Autodesk Fusion 360 part; units mm, degrees
(part 2 of 3)
sketch "Sketch2 (2)" plane through (0, 0, 0) normal (-1, 0, 0) x (0, -1, 0) in component "left"
  line L0 (-22.5, 130) -> (-22.5, 127)
  line L1 (-22.5, 127) -> (-32.1429, 127)
  line L2 (-32.1429, 127) -> (-32.1429, 130)
  line L3 (-32.1429, 130) -> (-42.8571, 130)
  line L4 (-42.8571, 130) -> (-42.8571, 127)
  line L5 (-42.8571, 127) -> (-52.5, 127)
  line L6 (-52.5, 127) -> (-52.5, 130)
  line L7 (-52.5, 130) -> (-52.5, 200)
  line L8 (-52.5, 200) -> (-72, 200)
  line L9 (-72, 200) -> (-72, 177.7778)
  line L10 (-72, 177.7778) -> (-75, 177.7778)
  line L11 (-75, 177.7778) -> (-75, 155.5556)
  line L12 (-75, 155.5556) -> (-72, 155.5556)
  line L13 (-72, 155.5556) -> (-72, 133.3333)
  line L14 (-72, 133.3333) -> (-75, 133.3333)
  line L15 (-75, 133.3333) -> (-75, 111.1111)
  line L16 (-75, 111.1111) -> (-72, 111.1111)
  line L17 (-72, 111.1111) -> (-72, 88.8889)
  line L18 (-72, 88.8889) -> (-75, 88.8889)
  line L19 (-75, 88.8889) -> (-75, 66.6667)
  line L20 (-75, 66.6667) -> (-72, 66.6667)
  line L21 (-72, 66.6667) -> (-72, 44.4444)
  line L22 (-72, 44.4444) -> (-75, 44.4444)
  line L23 (-75, 44.4444) -> (-75, 22.2222)
  line L24 (-75, 22.2222) -> (-72, 22.2222)
  line L25 (-72, 22.2222) -> (-72, 3)
  line L26 (-72, 3) -> (-64.2857, 3)
  line L27 (-64.2857, 3) -> (-64.2857, 0)
  line L28 (-64.2857, 0) -> (-53.5714, 0)
  line L29 (-53.5714, 0) -> (-53.5714, 3)
  line L30 (-53.5714, 3) -> (-42.8571, 3)
  line L31 (-42.8571, 3) -> (-42.8571, 0)
  line L32 (-42.8571, 0) -> (-32.1429, 0)
  line L33 (-32.1429, 0) -> (-32.1429, 3)
  line L34 (-32.1429, 3) -> (-21.4286, 3)
  line L35 (-21.4286, 3) -> (-21.4286, 0)
  line L36 (-21.4286, 0) -> (-10.7143, 0)
  line L37 (-10.7143, 0) -> (-10.7143, 3)
  line L38 (-10.7143, 3) -> (-3, 3)
  line L39 (-3, 3) -> (-3, 22.2222)
  line L40 (-3, 22.2222) -> (0, 22.2222)
  line L41 (0, 22.2222) -> (0, 44.4444)
  line L42 (0, 44.4444) -> (-3, 44.4444)
  line L43 (-3, 44.4444) -> (-3, 66.6667)
  line L44 (-3, 66.6667) -> (0, 66.6667)
  line L45 (0, 66.6667) -> (0, 88.8889)
  line L46 (0, 88.8889) -> (-3, 88.8889)
  line L47 (-3, 88.8889) -> (-3, 111.1111)
  line L48 (-3, 111.1111) -> (0, 111.1111)
  line L49 (0, 111.1111) -> (0, 133.3333)
  line L50 (0, 133.3333) -> (-3, 133.3333)
  line L51 (-3, 133.3333) -> (-3, 155.5556)
  line L52 (-3, 155.5556) -> (0, 155.5556)
  line L53 (0, 155.5556) -> (0, 177.7778)
  line L54 (0, 177.7778) -> (-3, 177.7778)
  line L55 (-3, 177.7778) -> (-3, 200)
  line L56 (-3, 200) -> (-22.5, 200)
  line L57 (-22.5, 200) -> (-22.5, 130)
  line L58 (-52.5, 200) -> (-22.5, 200)
  line L59 (-22.5, 200) -> (-22.5, 156)
  line L60 (-22.5, 156) -> (-52.5, 156)
  line L61 (-52.5, 156) -> (-52.5, 200)
  dimension "d161" = 26
  constraint horizontal L58
  constraint vertical L59
  constraint horizontal L60
  constraint vertical L61
  constraint coincident L57 L59.end
  constraint coincident L7.end L8.start
  measures "d161" distance of L3 L60
extrude "Extrude4'''" add sketch "Sketch2 (2)" against normal blind 3 contours L7 L57 L58 L59 L60 L61 bodies 5 in component "left"
combine "Combine6" operation cut target body 4 tool bodies 8 keep tools in component "right"
sketch "Sketch3 (2)" plane through (0, 0, 0) normal (-1, 0, 0) x (0, -1, 0) in component "left"
  line L0 (-22.5, 156) -> (-22.5, 130)
  line L1 (-22.5, 130) -> (-22.5, 127)
  line L2 (-22.5, 127) -> (-32.1429, 127)
  line L3 (-32.1429, 127) -> (-32.1429, 130)
  line L4 (-32.1429, 130) -> (-42.8571, 130)
  line L5 (-42.8571, 130) -> (-42.8571, 127)
  line L6 (-42.8571, 127) -> (-52.5, 127)
  line L7 (-52.5, 127) -> (-52.5, 130)
  line L8 (-52.5, 130) -> (-52.5, 156)
  line L9 (-52.5, 156) -> (-22.5, 156)
  line L10 (-3, 200) -> (-72, 200)
  line L11 (-72, 200) -> (-72, 177.7778)
  line L12 (-72, 177.7778) -> (-75, 177.7778)
  line L13 (-75, 177.7778) -> (-75, 155.5556)
  line L14 (-75, 155.5556) -> (-72, 155.5556)
  line L15 (-72, 155.5556) -> (-72, 133.3333)
  line L16 (-72, 133.3333) -> (-75, 133.3333)
  line L17 (-75, 133.3333) -> (-75, 111.1111)
  line L18 (-75, 111.1111) -> (-72, 111.1111)
  line L19 (-72, 111.1111) -> (-72, 88.8889)
  line L20 (-72, 88.8889) -> (-75, 88.8889)
  line L21 (-75, 88.8889) -> (-75, 66.6667)
  line L22 (-75, 66.6667) -> (-72, 66.6667)
  line L23 (-72, 66.6667) -> (-72, 44.4444)
  line L24 (-72, 44.4444) -> (-75, 44.4444)
  line L25 (-75, 44.4444) -> (-75, 22.2222)
  line L26 (-75, 22.2222) -> (-72, 22.2222)
  line L27 (-72, 22.2222) -> (-72, 3)
  line L28 (-72, 3) -> (-64.2857, 3)
  line L29 (-64.2857, 3) -> (-64.2857, 0)
  line L30 (-64.2857, 0) -> (-53.5714, 0)
  line L31 (-53.5714, 0) -> (-53.5714, 3)
  line L32 (-53.5714, 3) -> (-42.8571, 3)
  line L33 (-42.8571, 3) -> (-42.8571, 0)
  line L34 (-42.8571, 0) -> (-32.1429, 0)
  line L35 (-32.1429, 0) -> (-32.1429, 3)
  line L36 (-32.1429, 3) -> (-21.4286, 3)
  line L37 (-21.4286, 3) -> (-21.4286, 0)
  line L38 (-21.4286, 0) -> (-10.7143, 0)
  line L39 (-10.7143, 0) -> (-10.7143, 3)
  line L40 (-10.7143, 3) -> (-3, 3)
  line L41 (-3, 3) -> (-3, 22.2222)
  line L42 (-3, 22.2222) -> (0, 22.2222)
  line L43 (0, 22.2222) -> (0, 44.4444)
  line L44 (0, 44.4444) -> (-3, 44.4444)
  line L45 (-3, 44.4444) -> (-3, 66.6667)
  line L46 (-3, 66.6667) -> (0, 66.6667)
  line L47 (0, 66.6667) -> (0, 88.8889)
  line L48 (0, 88.8889) -> (-3, 88.8889)
  line L49 (-3, 88.8889) -> (-3, 111.1111)
  line L50 (-3, 111.1111) -> (0, 111.1111)
  line L51 (0, 111.1111) -> (0, 133.3333)
  line L52 (0, 133.3333) -> (-3, 133.3333)
  line L53 (-3, 133.3333) -> (-3, 155.5556)
  line L54 (-3, 155.5556) -> (0, 155.5556)
  line L55 (0, 155.5556) -> (0, 177.7778)
  line L56 (0, 177.7778) -> (-3, 177.7778)
  line L57 (-3, 177.7778) -> (-3, 200)
  circle A0 centre (-60, 117) radius 2.5
  dimension "d164" = 10
  dimension "d165" = 5
  dimension "d166" = 15
  measures "d164" distance of L6 A0.centre
  measures "d165" diameter of A0
  measures "d166" distance of L17 A0.centre
extrude "Extrude5'''" cut sketch "Sketch3 (2)" against normal blind 3 contours A0 bodies 5 in component "left"
sketch "Sketch7" plane through (75, 0, 0) normal (1, 0, 0) x (0, 1, 0) in component "right"
  line L0 (72, 78) -> (72, 66.6667)
  line L1 (72, 66.6667) -> (75, 66.6667)
  line L2 (75, 66.6667) -> (75, 88.8889)
  line L3 (75, 88.8889) -> (72, 88.8889)
  line L4 (72, 88.8889) -> (72, 111.1111)
  line L5 (72, 111.1111) -> (75, 111.1111)
  line L6 (75, 111.1111) -> (75, 133.3333)
  line L7 (75, 133.3333) -> (72, 133.3333)
  line L8 (72, 133.3333) -> (72, 155.5556)
  line L9 (72, 155.5556) -> (75, 155.5556)
  line L10 (75, 155.5556) -> (75, 177.7778)
  line L11 (75, 177.7778) -> (72, 177.7778)
  line L12 (72, 177.7778) -> (72, 200)
  line L13 (72, 200) -> (3, 200)
  line L14 (3, 200) -> (3, 177.7778)
  line L15 (3, 177.7778) -> (0, 177.7778)
  line L16 (0, 177.7778) -> (0, 155.5556)
  line L17 (0, 155.5556) -> (3, 155.5556)
  line L18 (3, 155.5556) -> (3, 133.3333)
  line L19 (3, 133.3333) -> (0, 133.3333)
  line L20 (0, 133.3333) -> (0, 111.1111)
  line L21 (0, 111.1111) -> (3, 111.1111)
  line L22 (3, 111.1111) -> (3, 88.8889)
  line L23 (3, 88.8889) -> (0, 88.8889)
  line L24 (0, 88.8889) -> (0, 66.6667)
  line L25 (0, 66.6667) -> (3, 66.6667)
  line L26 (3, 66.6667) -> (3, 44.4444)
  line L27 (3, 44.4444) -> (0, 44.4444)
  line L28 (0, 44.4444) -> (0, 22.2222)
  line L29 (0, 22.2222) -> (3, 22.2222)
  line L30 (3, 22.2222) -> (3, 3)
  line L31 (3, 3) -> (10.7143, 3)
  line L32 (10.7143, 3) -> (10.7143, 0)
  line L33 (10.7143, 0) -> (21.4286, 0)
  line L34 (21.4286, 0) -> (21.4286, 3)
  line L35 (21.4286, 3) -> (32.1429, 3)
  line L36 (32.1429, 3) -> (32.1429, 0)
  line L37 (32.1429, 0) -> (42.8571, 0)
  line L38 (42.8571, 0) -> (42.8571, 3)
  line L39 (42.8571, 3) -> (53.5714, 3)
  line L40 (53.5714, 3) -> (53.5714, 0)
  line L41 (53.5714, 0) -> (64.2857, 0)
  line L42 (64.2857, 0) -> (64.2857, 3)
  line L43 (64.2857, 3) -> (69, 3)
  line L44 (69, 3) -> (69, 78)
  line L45 (69, 78) -> (72, 78)
  circle A0 centre (60, 117) radius 2.5
  line L46 (52.5, 127) -> (42.8571, 127)
  line L47 (75, 0) -> (75, 200)
  dimension "d171" = 5
  dimension "d190" = 10
  dimension "d191" = 15
  measures "d171" diameter of A0
  measures "d190" distance of A0.centre L46
  measures "d191" distance of A0.centre L47
extrude "Extrude8" cut sketch "Sketch7" against normal blind 8 contours A0 bodies 4 in component "right"
sketch "Sketch3 (3)" plane through (0, 0, 0) normal (0, -1, 0) x (1, 0, 0) in component "front"
  line L0 (52.5, 156) -> (52.5, 130)
  line L1 (52.5, 130) -> (50, 130)
  line L2 (50, 130) -> (50, 127)
  line L3 (50, 127) -> (41.6667, 127)
  line L4 (41.6667, 127) -> (41.6667, 130)
  line L5 (41.6667, 130) -> (33.3333, 130)
  line L6 (33.3333, 130) -> (33.3333, 127)
  line L7 (33.3333, 127) -> (25, 127)
  line L8 (25, 127) -> (25, 130)
  line L9 (25, 130) -> (22.5, 130)
  line L10 (22.5, 130) -> (22.5, 156)
  line L11 (22.5, 156) -> (52.5, 156)
  line L12 (75, 200) -> (0, 200)
  line L13 (0, 200) -> (0, 177.7778)
  line L14 (0, 177.7778) -> (3, 177.7778)
  line L15 (3, 177.7778) -> (3, 155.5556)
  line L16 (3, 155.5556) -> (0, 155.5556)
  line L17 (0, 155.5556) -> (0, 133.3333)
  line L18 (0, 133.3333) -> (3, 133.3333)
  line L19 (3, 133.3333) -> (3, 111.1111)
  line L20 (3, 111.1111) -> (0, 111.1111)
  line L21 (0, 111.1111) -> (0, 88.8889)
  line L22 (0, 88.8889) -> (3, 88.8889)
  line L23 (3, 88.8889) -> (3, 66.6667)
  line L24 (3, 66.6667) -> (0, 66.6667)
  line L25 (0, 66.6667) -> (0, 44.4444)
  line L26 (0, 44.4444) -> (3, 44.4444)
  line L27 (3, 44.4444) -> (3, 22.2222)
  line L28 (3, 22.2222) -> (0, 22.2222)
  line L29 (0, 22.2222) -> (0, 3)
  line L30 (0, 3) -> (8.3333, 3)
  line L31 (8.3333, 3) -> (8.3333, 0)
  line L32 (8.3333, 0) -> (16.6667, 0)
  line L33 (16.6667, 0) -> (16.6667, 3)
  line L34 (16.6667, 3) -> (25, 3)
  line L35 (25, 3) -> (25, 0)
  line L36 (25, 0) -> (33.3333, 0)
  line L37 (33.3333, 0) -> (33.3333, 3)
  line L38 (33.3333, 3) -> (41.6667, 3)
  line L39 (41.6667, 3) -> (41.6667, 0)
  line L40 (41.6667, 0) -> (50, 0)
  line L41 (50, 0) -> (50, 3)
  line L42 (50, 3) -> (58.3333, 3)
  line L43 (58.3333, 3) -> (58.3333, 0)
  line L44 (58.3333, 0) -> (66.6667, 0)
  line L45 (66.6667, 0) -> (66.6667, 3)
  line L46 (66.6667, 3) -> (75, 3)
  line L47 (75, 3) -> (75, 22.2222)
  line L48 (75, 22.2222) -> (72, 22.2222)
  line L49 (72, 22.2222) -> (72, 44.4444)
  line L50 (72, 44.4444) -> (75, 44.4444)
  line L51 (75, 44.4444) -> (75, 66.6667)
  line L52 (75, 66.6667) -> (72, 66.6667)
  line L53 (72, 66.6667) -> (72, 88.8889)
  line L54 (72, 88.8889) -> (75, 88.8889)
  line L55 (75, 88.8889) -> (75, 111.1111)
  line L56 (75, 111.1111) -> (72, 111.1111)
  line L57 (72, 111.1111) -> (72, 133.3333)
  line L58 (72, 133.3333) -> (75, 133.3333)
  line L59 (75, 133.3333) -> (75, 155.5556)
  line L60 (75, 155.5556) -> (72, 155.5556)
  line L61 (72, 155.5556) -> (72, 177.7778)
  line L62 (72, 177.7778) -> (75, 177.7778)
  line L63 (75, 177.7778) -> (75, 200)
  circle A0 centre (18, 117) radius 2.5
  dimension "d174" = 10
  dimension "d175" = 15
  dimension "d176" = 5
  measures "d174" distance of L7 A0.centre
  measures "d175" distance of L19 A0.centre
  measures "d176" diameter of A0
extrude "Extrude5''''" cut sketch "Sketch3 (3)" against normal blind 3 contours A0 bodies 3 in component "front"
sketch "Sketch6 (2)" plane through (0, 72, 0) normal (0, -1, 0) x (1, 0, 0) in component "back"
  line L0 (13, 8) -> (13, 78)
  line L1 (13, 78) -> (62, 78)
  line L2 (62, 78) -> (62, 8)
  line L3 (62, 8) -> (13, 8)
  line L4 (0, 3) -> (8.3333, 3)
  line L5 (8.3333, 3) -> (8.3333, 0)
  line L6 (8.3333, 0) -> (16.6667, 0)
  line L7 (16.6667, 0) -> (16.6667, 3)
  line L8 (16.6667, 3) -> (25, 3)
  line L9 (25, 3) -> (25, 0)
  line L10 (25, 0) -> (33.3333, 0)
  line L11 (33.3333, 0) -> (33.3333, 3)
  line L12 (33.3333, 3) -> (41.6667, 3)
  line L13 (41.6667, 3) -> (41.6667, 0)
  line L14 (41.6667, 0) -> (50, 0)
  line L15 (50, 0) -> (50, 3)
  line L16 (50, 3) -> (58.3333, 3)
  line L17 (58.3333, 3) -> (58.3333, 0)
  line L18 (58.3333, 0) -> (66.6667, 0)
  line L19 (66.6667, 0) -> (66.6667, 3)
  line L20 (66.6667, 3) -> (75, 3)
  line L21 (75, 3) -> (75, 22.2222)
  line L22 (75, 22.2222) -> (75, 44.4444)
  line L23 (75, 44.4444) -> (75, 66.6667)
  line L24 (75, 66.6667) -> (72, 66.6667)
  line L25 (72, 66.6667) -> (72, 88.8889)
  line L26 (72, 88.8889) -> (75, 88.8889)
  line L27 (75, 88.8889) -> (75, 111.1111)
  line L28 (75, 111.1111) -> (72, 111.1111)
  line L29 (72, 111.1111) -> (72, 133.3333)
  line L30 (72, 133.3333) -> (75, 133.3333)
  line L31 (75, 133.3333) -> (75, 155.5556)
  line L32 (75, 155.5556) -> (72, 155.5556)
  line L33 (72, 155.5556) -> (72, 177.7778)
  line L34 (72, 177.7778) -> (75, 177.7778)
  line L35 (75, 177.7778) -> (75, 200)
  line L36 (75, 200) -> (0, 200)
  line L37 (0, 200) -> (0, 177.7778)
  line L38 (0, 177.7778) -> (3, 177.7778)
  line L39 (3, 177.7778) -> (3, 155.5556)
  line L40 (3, 155.5556) -> (0, 155.5556)
  line L41 (0, 155.5556) -> (0, 133.3333)
  line L42 (0, 133.3333) -> (3, 133.3333)
  line L43 (3, 133.3333) -> (3, 111.1111)
  line L44 (3, 111.1111) -> (0, 111.1111)
  line L45 (0, 111.1111) -> (0, 88.8889)
  line L46 (0, 88.8889) -> (3, 88.8889)
  line L47 (3, 88.8889) -> (3, 66.6667)
  line L48 (3, 66.6667) -> (0, 66.6667)
  line L49 (0, 66.6667) -> (0, 44.4444)
  line L50 (0, 44.4444) -> (3, 44.4444)
  line L51 (3, 44.4444) -> (3, 22.2222)
  line L52 (3, 22.2222) -> (0, 22.2222)
  line L53 (0, 22.2222) -> (0, 3)
  circle A0 centre (37.5, 117) radius 2.5
  line L54 (3, 127) -> (72, 127)
  line L55 (37.5, 117) -> (37.5, 127)
  dimension "d183" = 5
  dimension "d186" = 10
  constraint coincident A0.centre L55.start
  constraint coincident L54 L55.end
  constraint perpendicular L54 L55
  constraint midpoint L54 L55.end
  measures "d183" diameter of A0
  measures "d186" distance of A0.centre L55.end
extrude "Extrude7'" cut sketch "Sketch6 (2)" against normal blind 6 contours A0 bodies 2 in component "back"
extrude "Extrude9" cut sketch "spout_cut" against normal blind 10 contours L30 L48 L49 L50 L51 bodies 4 in component "right"
sketch "Sketch8" plane through (75, 0, 0) normal (1, 0, 0) x (0, 1, 0) in component "right"
  line L0 (52.5, 156) -> (22.5, 156)
  line L1 (22.5, 156) -> (22.5, 200)
  line L2 (22.5, 200) -> (52.5, 200)
  line L3 (52.5, 200) -> (52.5, 156)
  line L4 (22.5, 156) -> (52.5, 156)
  line L5 (52.5, 200) -> (52.5, 130)
  point P0 (22.5, 200)
  constraint horizontal L0
  constraint vertical L1
  constraint horizontal L2
  constraint vertical L3
  constraint coincident P0 L1.end
  constraint coincident L0.start L4
  constraint coincident L2.end L5
extrude "Extrude10" add sketch "Sketch8" against normal blind 3 bodies 4 in component "right"
combine "Combine7" operation cut target body 4 tool bodies 6 keep tools in component "right"
sketch "Sketch1 (5)" plane through (0, 0, 200) normal (0, 0, 1) x (-1, 0, 0) in component "cover"
  line L0 (-75, -75) -> (0, -75)
  line L1 (0, -75) -> (0, -72)
  line L2 (0, -72) -> (-75, -72)
  line L3 (-75, -72) -> (-75, -75)
  line L4 (-75, -75) -> (0, -75)
  line L5 (0, -75) -> (0, 0)
  line L6 (0, 0) -> (-75, 0)
  line L7 (-75, 0) -> (-75, -75)
  line L8 (5, 5) -> (-80, 5)
  line L9 (-80, 5) -> (-80, -80)
  line L10 (-80, -80) -> (5, -80)
  line L11 (5, -80) -> (5, 5)
  line L12 (0, -64.2857) -> (-3, -64.2857)
  line L13 (-3, -64.2857) -> (-3, -53.5714)
  line L14 (-3, -53.5714) -> (0, -53.5714)
  line L15 (0, -53.5714) -> (0, -64.2857)
  line L16 (0, -64.2857) -> (-3, -64.2857)
  line L17 (-3, -53.5714) -> (0, -53.5714)
  line L18 (-3, -42.8571) -> (0, -42.8571)
  line L19 (0, -42.8571) -> (0, -32.1429)
  line L20 (0, -32.1429) -> (-3, -32.1429)
  line L21 (-3, -32.1429) -> (-3, -42.8571)
  line L22 (-3, -21.4286) -> (0, -21.4286)
  line L23 (0, -21.4286) -> (0, -10.7143)
  line L24 (0, -10.7143) -> (-3, -10.7143)
  line L25 (-3, -10.7143) -> (-3, -21.4286)
  line L26 (0, -21.4286) -> (-3, -21.4286)
  line L27 (-3, -32.1429) -> (0, -32.1429)
  line L28 (-16.6667, -75) -> (-8.3333, -75)
  line L29 (-8.3333, -75) -> (-8.3333, -72)
  line L30 (-8.3333, -72) -> (-16.6667, -72)
  line L31 (-16.6667, -72) -> (-16.6667, -75)
  line L32 (-33.3333, -75) -> (-25, -75)
  line L33 (-25, -75) -> (-25, -72)
  line L34 (-25, -72) -> (-33.3333, -72)
  line L35 (-33.3333, -72) -> (-33.3333, -75)
  line L36 (-50, -75) -> (-41.6667, -75)
  line L37 (-41.6667, -75) -> (-41.6667, -72)
  line L38 (-41.6667, -72) -> (-50, -72)
  line L39 (-50, -72) -> (-50, -75)
  line L40 (-66.6667, -75) -> (-58.3333, -75)
  line L41 (-58.3333, -75) -> (-58.3333, -72)
  line L42 (-58.3333, -72) -> (-66.6667, -72)
  line L43 (-66.6667, -72) -> (-66.6667, -75)
  line L44 (-8.3333, -72) -> (-8.3333, -75)
  line L45 (-16.6667, -75) -> (-16.6667, -72)
  line L46 (-25, -72) -> (-25, -75)
  line L47 (-33.3333, -75) -> (-33.3333, -72)
  line L48 (-41.6667, -72) -> (-41.6667, -75)
  line L49 (-58.3333, -72) -> (-58.3333, -75)
  line L50 (-66.6667, -75) -> (-66.6667, -72)
  line L51 (5, -37.5) -> (-80, -37.5) construction
  line L52 (-37.5, -80) -> (-37.5, 5) construction
  line L53 (-72, -42.8571) -> (-75, -42.8571)
  line L54 (-75, -21.4286) -> (-75, -10.7143)
  line L55 (-72, -64.2857) -> (-72, -53.5714)
  line L56 (-75, -64.2857) -> (-72, -64.2857)
  line L57 (-72, -32.1429) -> (-72, -42.8571)
  line L58 (-75, -42.8571) -> (-75, -32.1429)
  line L59 (-72, -53.5714) -> (-75, -53.5714)
  line L60 (-75, -64.2857) -> (-72, -64.2857)
  line L61 (-72, -32.1429) -> (-75, -32.1429)
  line L62 (-75, -32.1429) -> (-72, -32.1429)
  line L63 (-75, -10.7143) -> (-72, -10.7143)
  line L64 (-72, -53.5714) -> (-75, -53.5714)
  line L65 (-75, -75) -> (-75, 0)
  line L66 (-75, -53.5714) -> (-75, -64.2857)
  line L67 (-80, -37.5) -> (5, -37.5) construction
  line L68 (-72, -10.7143) -> (-72, -21.4286)
  line L69 (-72, -21.4286) -> (-75, -21.4286)
  line L70 (-75, -21.4286) -> (-72, -21.4286)
  line L71 (-16.6667, -3) -> (-16.6667, 0)
  line L72 (-16.6667, 0) -> (-8.3333, 0)
  line L73 (-33.3333, -3) -> (-33.3333, 0)
  line L74 (-50, 0) -> (-41.6667, 0)
  line L75 (-8.3333, -3) -> (-16.6667, -3)
  line L76 (-41.6667, -3) -> (-50, -3)
  line L77 (-58.3333, 0) -> (-58.3333, -3)
  line L78 (-41.6667, -3) -> (-41.6667, 0)
  line L79 (-58.3333, -3) -> (-66.6667, -3)
  line L80 (-33.3333, 0) -> (-25, 0)
  line L81 (-25, 0) -> (-25, -3)
  line L82 (-8.3333, 0) -> (-8.3333, -3)
  line L83 (-8.3333, -3) -> (-8.3333, 0)
  line L84 (-66.6667, -3) -> (-66.6667, 0)
  line L85 (-66.6667, 0) -> (-58.3333, 0)
  line L86 (-25, -3) -> (-25, 0)
  line L87 (-66.6667, 0) -> (-66.6667, -3)
  line L88 (-25, -3) -> (-33.3333, -3)
  line L89 (-58.3333, -3) -> (-58.3333, 0)
  line L90 (-41.6667, 0) -> (-41.6667, -3)
  line L91 (-16.6667, 0) -> (-16.6667, -3)
  line L92 (-50, -3) -> (-50, 0)
  line L93 (-33.3333, 0) -> (-33.3333, -3)
  point P0 (-3, -42.8571)
  point P1 (-3, -10.7143)
  point P2 (-50, -72)
  point P3 (-72, -42.8571)
  point P4 (-72, -10.7143)
  point P5 (-50, -3)
  dimension "d199" = 5
  constraint horizontal L4
  constraint vertical L5
  constraint horizontal L6
  constraint vertical L7
  constraint coincident L5.end L6.start
  constraint coincident L0.start L3.end
  constraint horizontal L12
  constraint vertical L13
  constraint horizontal L14
  constraint vertical L15
  constraint coincident L5 L12.start
  constraint coincident L12.end L16
  constraint coincident L13.end L17
  constraint horizontal L18
  constraint vertical L19
  constraint horizontal L20
  constraint vertical L21
  constraint horizontal L22
  constraint vertical L23
  constraint horizontal L24
  constraint vertical L25
  constraint coincident L5 L23.end
  constraint coincident L22.start L26
  constraint coincident L20.end L27
  constraint coincident P0 L18.start
  constraint coincident L13 L12.end
  constraint coincident P1 L24.end
  constraint horizontal L28
  constraint vertical L29
  constraint horizontal L30
  constraint vertical L31
  constraint coincident L2 L29.end
  constraint coincident L4 L28.start
  constraint horizontal L32
  constraint vertical L33
  constraint horizontal L34
  constraint vertical L35
  constraint coincident L2 L33.end
  constraint coincident L4 L32.start
  constraint horizontal L36
  constraint vertical L37
  constraint horizontal L38
  constraint vertical L39
  constraint coincident L2 L37.end
  constraint coincident L4 L36.start
  constraint horizontal L40
  constraint vertical L41
  constraint horizontal L42
  constraint vertical L43
  constraint coincident L2 L41.end
  constraint coincident L4 L40.start
  constraint coincident L29.end L44
  constraint coincident L30.end L45
  constraint coincident L33.end L46
  constraint coincident L34.end L47
  constraint coincident L37.end L48
  constraint coincident L39 P2
  constraint coincident L41.end L49
  constraint coincident L42.end L50
  constraint midpoint L11 L51.start
  constraint midpoint L9 L51.end
  constraint midpoint L10 L52.start
  constraint midpoint L8 L52.end
  constraint symmetric L0.end L52 L0.start
  constraint symmetric L5.end L52 L6.end
  constraint symmetric L12.start L52 L56.start
  constraint symmetric L12.end L52 L55.start
  constraint symmetric L13.end L52 L55.end
  constraint symmetric L14.end L52 L59.end
  constraint symmetric P0 L52 P3
  constraint symmetric L18.end L52 L53.end
  constraint symmetric L19.end L52 L58.end
  constraint symmetric L20.end L52 L57.start
  constraint symmetric L22.start L52 L68.end
  constraint symmetric L22.end L52 L54.start
  constraint symmetric L23.end L52 L54.end
  constraint symmetric P1 L52 P4
  constraint symmetric L51.start L52 L51.end
  constraint symmetric L51.end L52 L51.start
  constraint symmetric L28.start L51 L71.end
  constraint symmetric L28.end L51 L72.end
  constraint symmetric L29.end L51 L75.start
  constraint symmetric L30.end L51 L71.start
  constraint symmetric L32.start L51 L73.end
  constraint symmetric L32.end L51 L80.end
  constraint symmetric L33.end L51 L81.end
  constraint symmetric L34.end L51 L73.start
  constraint symmetric L36.start L51 L74.start
  constraint symmetric L36.end L51 L74.end
  constraint symmetric L37.end L51 L76.start
  constraint symmetric P2 L51 P5
  constraint symmetric L40.start L51 L84.end
  constraint symmetric L40.end L51 L77.start
  constraint symmetric L41.end L51 L77.end
  constraint symmetric L42.end L51 L79.end
extrude "Extrude1'''''''" add sketch "Sketch1 (5)" against normal blind 3 separate body contours L0 L2 L3 L4 L7 L43 L50 L65 | L2 L5 L6 L7 L12 L13 L14 L16 L17 L18 L20 L21 L22 L24 L25 L26 L27 L30 L34 L38 L42 L53 L55 L56 L57 L59 L60 L61 L62 L63 L64 L65 L68 L69 L70 L71 L73 L75 L76 L77 L78 L79 L81 L82 L83 L84 L86 L87 L88 L89 L90 L91 L92 L93 | L0 L2 L4 L39 L41 L49 | L0 L2 L4 L35 L37 L47 L48 | L0 L2 L4 L31 L33 L45 L46 | L0 L1 L2 L4 L5 L29 L44 | L8 L9 L10 L11 makes body 9 in component "cover"
combine "Combine5'" operation cut target body 3 tool bodies 9 keep tools in component "front"
combine "Combine9" operation cut target body 4 tool bodies 9 keep tools in component "right"
combine "Combine5''" operation cut target body 2 tool bodies 9 keep tools in component "back"
combine "Combine4'" operation cut target body 5 tool bodies 9 keep tools in component "left"
sketch "Sketch7 (2)" plane through (0, 75, 0) normal (0, 1, 0) x (-1, 0, 0) in component "back"
  line L0 (-13, 78) -> (-13, 8)
  line L1 (-13, 8) -> (-62, 8)
  line L2 (-62, 8) -> (-62, 78)
  line L3 (-62, 78) -> (-13, 78)
  circle A0 centre (-37.5, 117) radius 2.5
  line L4 (0, 197) -> (-8.3333, 197)
  line L5 (-8.3333, 197) -> (-8.3333, 200)
  line L6 (-8.3333, 200) -> (-16.6667, 200)
  line L7 (-16.6667, 200) -> (-16.6667, 197)
  line L8 (-16.6667, 197) -> (-25, 197)
  line L9 (-25, 197) -> (-25, 200)
  line L10 (-25, 200) -> (-33.3333, 200)
  line L11 (-33.3333, 200) -> (-33.3333, 197)
  line L12 (-33.3333, 197) -> (-41.6667, 197)
  line L13 (-41.6667, 197) -> (-41.6667, 200)
  line L14 (-41.6667, 200) -> (-50, 200)
  line L15 (-50, 200) -> (-50, 197)
  line L16 (-50, 197) -> (-58.3333, 197)
  line L17 (-58.3333, 197) -> (-58.3333, 200)
  line L18 (-58.3333, 200) -> (-66.6667, 200)
  line L19 (-66.6667, 200) -> (-66.6667, 197)
  line L20 (-66.6667, 197) -> (-75, 197)
  line L21 (-75, 197) -> (-75, 177.7778)
  line L22 (-75, 177.7778) -> (-72, 177.7778)
  line L23 (-72, 177.7778) -> (-72, 155.5556)
  line L24 (-72, 155.5556) -> (-75, 155.5556)
  line L25 (-75, 155.5556) -> (-75, 133.3333)
  line L26 (-75, 133.3333) -> (-72, 133.3333)
  line L27 (-72, 133.3333) -> (-72, 111.1111)
  line L28 (-72, 111.1111) -> (-75, 111.1111)
  line L29 (-75, 111.1111) -> (-75, 88.8889)
  line L30 (-75, 88.8889) -> (-72, 88.8889)
  line L31 (-72, 88.8889) -> (-72, 66.6667)
  line L32 (-72, 66.6667) -> (-75, 66.6667)
  line L33 (-75, 66.6667) -> (-75, 44.4444)
  line L34 (-75, 44.4444) -> (-75, 22.2222)
  line L35 (-75, 22.2222) -> (-75, 3)
  line L36 (-75, 3) -> (-66.6667, 3)
  line L37 (-66.6667, 3) -> (-66.6667, 0)
  line L38 (-66.6667, 0) -> (-58.3333, 0)
  line L39 (-58.3333, 0) -> (-58.3333, 3)
  line L40 (-58.3333, 3) -> (-50, 3)
  line L41 (-50, 3) -> (-50, 0)
  line L42 (-50, 0) -> (-41.6667, 0)
  line L43 (-41.6667, 0) -> (-41.6667, 3)
  line L44 (-41.6667, 3) -> (-33.3333, 3)
  line L45 (-33.3333, 3) -> (-33.3333, 0)
  line L46 (-33.3333, 0) -> (-25, 0)
  line L47 (-25, 0) -> (-25, 3)
  line L48 (-25, 3) -> (-16.6667, 3)
  line L49 (-16.6667, 3) -> (-16.6667, 0)
  line L50 (-16.6667, 0) -> (-8.3333, 0)
  line L51 (-8.3333, 0) -> (-8.3333, 3)
  line L52 (-8.3333, 3) -> (0, 3)
  line L53 (0, 3) -> (0, 22.2222)
  line L54 (0, 22.2222) -> (-3, 22.2222)
  line L55 (-3, 22.2222) -> (-3, 44.4444)
  line L56 (-3, 44.4444) -> (0, 44.4444)
  line L57 (0, 44.4444) -> (0, 66.6667)
  line L58 (0, 66.6667) -> (-3, 66.6667)
  line L59 (-3, 66.6667) -> (-3, 88.8889)
  line L60 (-3, 88.8889) -> (0, 88.8889)
  line L61 (0, 88.8889) -> (0, 111.1111)
  line L62 (0, 111.1111) -> (-3, 111.1111)
  line L63 (-3, 111.1111) -> (-3, 133.3333)
  line L64 (-3, 133.3333) -> (0, 133.3333)
  line L65 (0, 133.3333) -> (0, 155.5556)
  line L66 (0, 155.5556) -> (-3, 155.5556)
  line L67 (-3, 155.5556) -> (-3, 177.7778)
  line L68 (-3, 177.7778) -> (0, 177.7778)
  line L69 (0, 177.7778) -> (0, 197)
  circle A1 centre (-37.5, 182) radius 5
  line L70 (-37.5, 197) -> (-37.5, 167)
  dimension "d202" = 10
  dimension "d203" = 15
  constraint midpoint L12 L70.start
  constraint perpendicular L12 L70
  constraint coincident A1.centre L70
  measures "d202" diameter of A1
  measures "d203" distance of L12 A1.centre
extrude "Extrude8'" cut sketch "Sketch7 (2)" against normal blind 6 contours A1 L70 | A1 L70 bodies 2 in component "back"
sketch "Sketch1 (6)" plane through (0, 0, 156) normal (0, 0, -1) x (1, 0, 0) in component "Main"
  line L0 (52.5, 0) -> (22.5, 0)
  line L1 (22.5, 0) -> (22.5, -3)
  line L2 (22.5, -3) -> (52.5, -3)
  line L3 (52.5, -3) -> (52.5, 0)
  line L4 (3, -3) -> (72, -3)
  line L5 (72, -3) -> (72, -72)
  line L6 (72, -72) -> (3, -72)
  line L7 (3, -72) -> (3, -3)
  point P0 (3, -3)
  point P1 (66.6667, -72)
  dimension "d206" = 69
  constraint horizontal L4
  constraint vertical L5
  constraint horizontal L6
  constraint vertical L7
  constraint coincident P0 L4.start
  constraint coincident L6 P1
  measures "d206" distance of P0 L4.end
extrude "Extrude1''''''''" add sketch "Sketch1 (6)" against normal blind 2 separate body contours L2 L4 L5 L6 L7 makes body 10 in component "Main"
sketch "Sketch2 (3)" plane through (0, 0, 158) normal (0, 0, 1) x (-1, 0, 0) in component "Main"
  line L0 (-72, -72) -> (-3, -72)
  line L1 (-3, -72) -> (-3, -3)
  line L2 (-3, -3) -> (-72, -3)
  line L3 (-72, -3) -> (-72, -72)
  line L4 (-37.5, -72) -> (-37.5, -3) construction
  line L5 (-3, -37.5) -> (-72, -37.5) construction
  line L6 (-31, -48.875) -> (-44, -48.875)
  line L7 (-44, -48.875) -> (-44, -26.125)
  line L8 (-44, -26.125) -> (-31, -26.125)
  line L9 (-31, -26.125) -> (-31, -48.875)
  line L10 (-31, -48.875) -> (-44, -26.125) construction
  line L11 (-44, -48.875) -> (-31, -26.125) construction
  line L12 (-22, -49.5) -> (-3, -49.5)
  line L13 (-3, -49.5) -> (-3, -25.5)
  line L14 (-3, -25.5) -> (-22, -25.5)
  line L15 (-22, -25.5) -> (-22, -49.5)
  line L16 (-17, -55.875) -> (-58, -55.875)
  line L17 (-58, -55.875) -> (-58, -72)
  line L18 (-58, -72) -> (-17, -72)
  line L19 (-17, -72) -> (-17, -55.875)
  line L20 (-72, -49.5) -> (-53, -49.5)
  line L21 (-53, -49.5) -> (-53, -25.5)
  line L22 (-53, -25.5) -> (-72, -25.5)
  line L23 (-72, -25.5) -> (-72, -49.5)
  line L24 (-49.5, -3) -> (-25.5, -3)
  line L25 (-25.5, -3) -> (-25.5, -16.125)
  line L26 (-25.5, -16.125) -> (-49.5, -16.125)
  line L27 (-49.5, -16.125) -> (-49.5, -3)
  point P0 (-37.5, -37.5)
  dimension "d233" = 13
  dimension "d234" = 22.75
  dimension "d236" = 14
  dimension "d237" = 7
  dimension "d238" = 9
  dimension "d239" = 24
  dimension "d240" = 10
  constraint midpoint L0 L4.start
  constraint midpoint L2 L4.end
  constraint midpoint L1 L5.start
  constraint midpoint L3 L5.end
  constraint horizontal L6
  constraint perpendicular L6 L7
  constraint parallel L6 L8
  constraint parallel L7 L9
  constraint coincident L10 P0
  constraint coincident L11 P0
  constraint midpoint L4 P0
  constraint horizontal L12
  constraint vertical L13
  constraint horizontal L14
  constraint vertical L15
  constraint horizontal L16
  constraint vertical L17
  constraint horizontal L18
  constraint vertical L19
  constraint horizontal L20
  constraint vertical L21
  constraint horizontal L22
  constraint vertical L23
  constraint horizontal L24
  constraint vertical L25
  constraint horizontal L26
  constraint vertical L27
  constraint midpoint L0 L18
  constraint midpoint L3 L23
  constraint midpoint L2 L24
  constraint midpoint L1 L13
  constraint equal L12 L20
  constraint equal L15 L26
  constraint equal L15 L21
  measures "d233" distance of L6.start L6.end
  measures "d234" distance of L6.end L7.end
  measures "d236" distance of L1 L19
  measures "d237" distance of L6 L16
  measures "d238" distance of L9 L15
  measures "d239" distance of L25.end L26.end
  measures "d240" distance of L8 L26
extrude "Extrude2'''''" cut sketch "Sketch2 (3)" against normal blind 7 contours L0 L16 L17 L18 L19 | L3 L20 L21 L22 L23 | L1 L12 L13 L14 L15 | L2 L24 L25 L26 L27 | L6 L7 L8 L9 bodies 10 in component "Main"
sketch "Sketch3 (4)" plane through (0, 0, 158) normal (0, 0, 1) x (-1, 0, 0) in component "Main"
  line L0 (-22, -25.5) -> (-3, -25.5)
  line L1 (-3, -25.5) -> (-3, -3)
  line L2 (-3, -3) -> (-25.5, -3)
  line L3 (-25.5, -3) -> (-25.5, -16.125)
  line L4 (-25.5, -16.125) -> (-49.5, -16.125)
  line L5 (-49.5, -16.125) -> (-49.5, -3)
  line L6 (-49.5, -3) -> (-72, -3)
  line L7 (-72, -3) -> (-72, -25.5)
  line L8 (-72, -25.5) -> (-53, -25.5)
  line L9 (-53, -25.5) -> (-53, -49.5)
  line L10 (-53, -49.5) -> (-72, -49.5)
  line L11 (-72, -49.5) -> (-72, -72)
  line L12 (-72, -72) -> (-58, -72)
  line L13 (-58, -72) -> (-58, -55.875)
  line L14 (-58, -55.875) -> (-17, -55.875)
  line L15 (-17, -55.875) -> (-17, -72)
  line L16 (-17, -72) -> (-3, -72)
  line L17 (-3, -72) -> (-3, -49.5)
  line L18 (-3, -49.5) -> (-22, -49.5)
  line L19 (-22, -49.5) -> (-22, -25.5)
  line L20 (-44, -48.875) -> (-44, -26.125)
  line L21 (-44, -26.125) -> (-31, -26.125)
  line L22 (-31, -26.125) -> (-31, -48.875)
  line L23 (-31, -48.875) -> (-44, -48.875)
  line L24 (-22, -49.5) -> (-24, -49.5)
  line L25 (-24, -49.5) -> (-24, -44.7)
  line L26 (-24, -44.7) -> (-22, -44.7)
  line L27 (-22, -44.7) -> (-22, -49.5)
  line L28 (-24, -44.7) -> (-22, -44.7)
  line L29 (-22, -44.7) -> (-22, -39.9)
  line L30 (-22, -39.9) -> (-24, -39.9)
  line L31 (-24, -39.9) -> (-24, -44.7)
  line L32 (-24, -39.9) -> (-22, -39.9)
  line L33 (-22, -39.9) -> (-22, -35.1)
  line L34 (-22, -35.1) -> (-24, -35.1)
  line L35 (-24, -35.1) -> (-24, -39.9)
  line L36 (-24, -35.1) -> (-22, -35.1)
  line L37 (-22, -35.1) -> (-22, -30.3)
  line L38 (-22, -30.3) -> (-24, -30.3)
  line L39 (-24, -30.3) -> (-24, -35.1)
  line L40 (-24, -30.3) -> (-22, -30.3)
  line L41 (-22, -30.3) -> (-22, -25.5)
  line L42 (-22, -25.5) -> (-24, -25.5)
  line L43 (-24, -25.5) -> (-24, -30.3)
  line L44 (-25.5, -16.125) -> (-30.3, -16.125)
  line L45 (-30.3, -16.125) -> (-30.3, -18.125)
  line L46 (-30.3, -18.125) -> (-25.5, -18.125)
  line L47 (-25.5, -18.125) -> (-25.5, -16.125)
  line L48 (-30.3, -18.125) -> (-35.1, -18.125)
  line L49 (-35.1, -18.125) -> (-35.1, -16.125)
  line L50 (-35.1, -16.125) -> (-30.3, -16.125)
  line L51 (-30.3, -16.125) -> (-30.3, -18.125)
  line L52 (-35.1, -18.125) -> (-39.9, -18.125)
  line L53 (-39.9, -18.125) -> (-39.9, -16.125)
  line L54 (-39.9, -16.125) -> (-35.1, -16.125)
  line L55 (-35.1, -16.125) -> (-35.1, -18.125)
  line L56 (-39.9, -18.125) -> (-44.7, -18.125)
  line L57 (-44.7, -18.125) -> (-44.7, -16.125)
  line L58 (-44.7, -16.125) -> (-39.9, -16.125)
  line L59 (-39.9, -16.125) -> (-39.9, -18.125)
  line L60 (-44.7, -18.125) -> (-49.5, -18.125)
  line L61 (-49.5, -18.125) -> (-49.5, -16.125)
  line L62 (-49.5, -16.125) -> (-44.7, -16.125)
  line L63 (-44.7, -16.125) -> (-44.7, -18.125)
  line L64 (-37.5, -72) -> (-37.5, -3)
  line L65 (-51, -49.5) -> (-51, -44.7)
  line L66 (-51, -35.1) -> (-53, -35.1)
  line L67 (-51, -44.7) -> (-53, -44.7)
  line L68 (-51, -35.1) -> (-51, -39.9)
  line L69 (-53, -49.5) -> (-51, -49.5)
  line L70 (-53, -30.3) -> (-51, -30.3)
  line L71 (-51, -39.9) -> (-51, -44.7)
  line L72 (-51, -25.5) -> (-51, -30.3)
  line L73 (-51, -44.7) -> (-53, -44.7)
  line L74 (-51, -39.9) -> (-53, -39.9)
  line L75 (-53, -39.9) -> (-51, -39.9)
  line L76 (-51, -30.3) -> (-53, -30.3)
  line L77 (-53, -35.1) -> (-51, -35.1)
  line L78 (-53, -25.5) -> (-51, -25.5)
  line L79 (-51, -30.3) -> (-51, -35.1)
  line L80 (-53, -44.7) -> (-53, -49.5)
  line L81 (-53, -44.7) -> (-53, -39.9)
  line L82 (-53, -39.9) -> (-53, -35.1)
  line L83 (-53, -35.1) -> (-53, -30.3)
  line L84 (-53, -30.3) -> (-53, -25.5)
  dimension "d243" = 2
  dimension "d244" = 4.8
  dimension "d245" = 4.8
  dimension "d246" = 4.8
  dimension "d247" = 4.8
  dimension "d248" = 4.8
  dimension "d249" = 2
  dimension "d250" = 4.8
  dimension "d251" = 4.8
  dimension "d252" = 4.8
  dimension "d253" = 4.8
  dimension "d254" = 4.8
  constraint horizontal L24
  constraint vertical L25
  constraint horizontal L26
  constraint vertical L27
  constraint coincident L18.end L19.start
  constraint horizontal L28
  constraint vertical L29
  constraint horizontal L30
  constraint vertical L31
  constraint coincident L19 L29.end
  constraint horizontal L32
  constraint vertical L33
  constraint horizontal L34
  constraint vertical L35
  constraint coincident L19 L33.end
  constraint horizontal L36
  constraint vertical L37
  constraint horizontal L38
  constraint vertical L39
  constraint coincident L19 L37.end
  constraint horizontal L40
  constraint vertical L41
  constraint horizontal L42
  constraint vertical L43
  constraint coincident L19 L0.start
  constraint horizontal L44
  constraint vertical L45
  constraint horizontal L46
  constraint vertical L47
  constraint coincident L3.end L4.start
  constraint horizontal L48
  constraint vertical L49
  constraint horizontal L50
  constraint vertical L51
  constraint coincident L4 L49.end
  constraint horizontal L52
  constraint vertical L53
  constraint horizontal L54
  constraint vertical L55
  constraint coincident L4 L53.end
  constraint horizontal L56
  constraint vertical L57
  constraint horizontal L58
  constraint vertical L59
  constraint coincident L4 L57.end
  constraint horizontal L60
  constraint vertical L61
  constraint horizontal L62
  constraint vertical L63
  constraint coincident L4 L5.start
  constraint symmetric L18.end L64 L9.end
  constraint symmetric L24.end L64 L65.start
  constraint symmetric L25.end L64 L65.end
  constraint symmetric L26.end L64 L67.end
  constraint symmetric L29.end L64 L74.end
  constraint symmetric L30.end L64 L68.end
  constraint symmetric L33.end L64 L66.end
  constraint symmetric L34.end L64 L66.start
  constraint symmetric L37.end L64 L70.start
  constraint symmetric L38.end L64 L70.end
  constraint symmetric L0.start L64 L8.end
  constraint symmetric L42.end L64 L72.start
  measures "d243" distance of L18.end L24.end
  measures "d244" distance of L24.end L25.end
  measures "d245" distance of L25.end L30.end
  measures "d246" distance of L30.end L34.end
  measures "d247" distance of L34.end L38.end
  measures "d248" distance of L38.end L42.end
  measures "d249" distance of L3.end L46.end
  measures "d250" distance of L45.end L46.end
  measures "d251" distance of L45.end L48.end
  measures "d252" distance of L48.end L52.end
  measures "d253" distance of L52.end L56.end
  measures "d254" distance of L56.end L60.end
extrude "Extrude3'''''" cut sketch "Sketch3 (4)" against normal blind 9 contours L19 L38 L40 L41 L42 L43 | L19 L30 L32 L33 L34 L35 L36 | L4 L44 L45 L46 L47 L51 | L19 L24 L25 L26 L27 L28 | L4 L49 L52 L54 L55 L64 | L4 L52 L53 L54 L59 L64 | L4 L57 L60 L61 L62 L63 | L9 L70 L72 L76 L78 L84 | L9 L65 L67 L69 L73 L80 | L9 L66 L68 L74 L75 L77 L82 bodies 10 in component "Main"
sketch "Sketch1 (7)" plane through (51, 0, 0) normal (1, 0, 0) x (0, 1, 0) in component "side right"
  line L0 (35.1, 156) -> (39.9, 156)
  line L1 (39.9, 156) -> (39.9, 158)
  line L2 (39.9, 158) -> (35.1, 158)
  line L3 (35.1, 158) -> (35.1, 156)
  line L4 (25.5, 158) -> (49.5, 158)
  line L5 (49.5, 158) -> (49.5, 151)
  line L6 (49.5, 151) -> (25.5, 151)
  line L7 (25.5, 151) -> (25.5, 158)
  point P0 (25.5, 158)
  point P1 (49.5, 158)
  dimension "d257" = 7
  constraint horizontal L4
  constraint vertical L5
  constraint horizontal L6
  constraint vertical L7
  constraint coincident P0 L4.start
  constraint coincident P1 L4.end
  measures "d257" distance of P1 L5.end
extrude "Extrude1'''''''''" add sketch "Sketch1 (7)" along normal blind 2 separate body makes body 11 in component "side right"
extrude "Extrude1''''''''''" add 1 faces at (53, 38.3, 153.3333) along direction (-1, 0, 0) blind 2 from surface at 29 separate body on bodies 11 makes body 12 in component "side left"
combine "Combine1'''''" operation cut target body 11 tool bodies 10 keep tools in component "side right"
combine "Combine1''''''" operation cut target body 12 tool bodies 10 keep tools in component "side left"
sketch "Sketch1 (8)" plane through (0, 18.125, 0) normal (0, -1, 0) x (1, 0, 0) in component "side front"
  line L0 (35.1, 156) -> (39.9, 156)
  line L1 (39.9, 156) -> (39.9, 158)
  line L2 (39.9, 158) -> (35.1, 158)
  line L3 (35.1, 158) -> (35.1, 156)
  line L4 (25.5, 158) -> (49.5, 158)
  line L5 (49.5, 158) -> (49.5, 151)
  line L6 (49.5, 151) -> (25.5, 151)
  line L7 (25.5, 151) -> (25.5, 158)
  point P0 (25.5, 158)
  point P1 (49.5, 158)
  dimension "d263" = 7
  constraint horizontal L4
  constraint vertical L5
  constraint horizontal L6
  constraint vertical L7
  constraint coincident P0 L4.start
  constraint coincident L5 P1
  measures "d263" distance of P1 L5.end
extrude "Extrude1'''''''''''" add sketch "Sketch1 (8)" along normal blind 2 separate body makes body 13 in component "side front"
combine "Combine1'''''''" operation cut target body 13 tool bodies 10 keep tools in component "side front"
sketch "Sketch4 (3)" plane through (0, 0, 158) normal (0, 0, 1) x (-1, 0, 0) in component "Main"
  line L0 (-51, -30.3) -> (-53, -30.3)
  line L1 (-53, -30.3) -> (-53, -35.1)
  line L2 (-53, -35.1) -> (-51, -35.1)
  line L3 (-51, -35.1) -> (-51, -39.9)
  line L4 (-51, -39.9) -> (-53, -39.9)
  line L5 (-53, -39.9) -> (-53, -44.7)
  line L6 (-53, -44.7) -> (-51, -44.7)
  line L7 (-51, -44.7) -> (-51, -49.5)
  line L8 (-51, -49.5) -> (-72, -49.5)
  line L9 (-72, -49.5) -> (-72, -72)
  line L10 (-72, -72) -> (-58, -72)
  line L11 (-58, -72) -> (-58, -55.875)
  line L12 (-58, -55.875) -> (-17, -55.875)
  line L13 (-17, -55.875) -> (-17, -72)
  line L14 (-17, -72) -> (-3, -72)
  line L15 (-3, -72) -> (-3, -49.5)
  line L16 (-3, -49.5) -> (-24, -49.5)
  line L17 (-24, -49.5) -> (-24, -44.7)
  line L18 (-24, -44.7) -> (-22, -44.7)
  line L19 (-22, -44.7) -> (-22, -39.9)
  line L20 (-22, -39.9) -> (-24, -39.9)
  line L21 (-24, -39.9) -> (-24, -35.1)
  line L22 (-24, -35.1) -> (-22, -35.1)
  line L23 (-22, -35.1) -> (-22, -30.3)
  line L24 (-22, -30.3) -> (-24, -30.3)
  line L25 (-24, -30.3) -> (-24, -25.5)
  line L26 (-24, -25.5) -> (-3, -25.5)
  line L27 (-3, -25.5) -> (-3, -3)
  line L28 (-3, -3) -> (-25.5, -3)
  line L29 (-25.5, -3) -> (-25.5, -18.125)
  line L30 (-25.5, -18.125) -> (-30.3, -18.125)
  line L31 (-30.3, -18.125) -> (-30.3, -16.125)
  line L32 (-30.3, -16.125) -> (-35.1, -16.125)
  line L33 (-35.1, -16.125) -> (-35.1, -18.125)
  line L34 (-35.1, -18.125) -> (-39.9, -18.125)
  line L35 (-39.9, -18.125) -> (-39.9, -16.125)
  line L36 (-39.9, -16.125) -> (-44.7, -16.125)
  line L37 (-44.7, -16.125) -> (-44.7, -18.125)
  line L38 (-44.7, -18.125) -> (-49.5, -18.125)
  line L39 (-49.5, -18.125) -> (-49.5, -3)
  line L40 (-49.5, -3) -> (-72, -3)
  line L41 (-72, -3) -> (-72, -25.5)
  line L42 (-72, -25.5) -> (-51, -25.5)
  line L43 (-51, -25.5) -> (-51, -30.3)
  line L44 (-44, -48.875) -> (-44, -26.125)
  line L45 (-44, -26.125) -> (-31, -26.125)
  line L46 (-31, -26.125) -> (-31, -48.875)
  line L47 (-31, -48.875) -> (-44, -48.875)
  line L48 (0, -64.5) -> (-3, -64.5)
  line L49 (-3, -64.5) -> (-3, -57)
  line L50 (-3, -57) -> (0, -57)
  line L51 (0, -57) -> (0, -64.5)
  line L52 (-3, -37.5) -> (-72, -37.5)
  line L53 (-3, -10.5) -> (-3, -18)
  line L54 (0, -10.5) -> (-3, -10.5)
  line L55 (0, -18) -> (0, -10.5)
  line L56 (-3, -18) -> (0, -18)
  line L57 (-37.5, -72) -> (-37.5, -3)
  line L58 (-75, -57) -> (-75, -64.5)
  line L59 (-72, -57) -> (-75, -57)
  line L60 (-75, -64.5) -> (-72, -64.5)
  line L61 (-72, -64.5) -> (-72, -57)
  line L62 (-72, -18) -> (-75, -18)
  line L63 (-75, -18) -> (-75, -10.5)
  line L64 (-75, -10.5) -> (-72, -10.5)
  line L65 (-72, -10.5) -> (-72, -18)
  circle A0 centre (-37.5, -51.6392) radius 1.1
  line L66 (-31, -48.875) -> (-44, -48.875)
  circle A1 centre (-37.5, -23.3608) radius 1.1
  dimension "d266" = 7.5
  dimension "d267" = 3
  dimension "d268" = 2.2
  dimension "d269" = 2.7642
  constraint horizontal L48
  constraint vertical L49
  constraint horizontal L50
  constraint vertical L51
  constraint midpoint L15 L49
  constraint symmetric L48.start L52 L54.start
  constraint symmetric L48.end L52 L53.start
  constraint symmetric L49.end L52 L53.end
  constraint symmetric L50.end L52 L55.start
  constraint symmetric L48.start L57 L58.end
  constraint symmetric L48.end L57 L60.end
  constraint symmetric L49.end L57 L59.start
  constraint symmetric L50.end L57 L58.start
  constraint symmetric L53.start L57 L64.end
  constraint symmetric L53.end L57 L62.start
  constraint symmetric L54.start L57 L63.end
  constraint symmetric L55.start L57 L62.end
  constraint coincident L57 A0.centre
  constraint symmetric L52 A0 A1
  measures "d266" distance of L48.start L50.end
  measures "d267" distance of L49.end L50.end
  measures "d268" diameter of A0
  measures "d269" distance of A0.centre L66
extrude "Extrude4''''" add sketch "Sketch4 (3)" against normal blind 2 contours L41 L62 L63 L64 L65 | L9 L58 L59 L60 L61 | L15 L48 L49 L50 L51 | L27 L53 L54 L55 L56 bodies 10 in component "Main"
extrude "Extrude5'''''" cut sketch "Sketch4 (3)" against normal blind 4 contours L57 A0 | L57 A0 | L57 A1 | L57 A1 bodies 10 in component "Main"
combine "Combine5'''" operation cut target body 5 tool bodies 10 keep tools in component "left"
combine "Combine10" operation cut target body 4 tool bodies 10 keep tools in component "right"
sketch "cover.dxf" plane through (0, 0, 200) normal (0, 0, 1) x (-1, 0, 0) in component "cover"
  line L0 (-25, 0) -> (-25, -3)
  line L1 (-25, -3) -> (-33.3333, -3)
  line L2 (-33.3333, -3) -> (-33.3333, 0)
  line L3 (-33.3333, 0) -> (-25, 0)
  line L4 (-8.3333, 0) -> (-8.3333, -3)
  line L5 (-8.3333, -3) -> (-16.6667, -3)
  line L6 (-16.6667, -3) -> (-16.6667, 0)
  line L7 (-16.6667, 0) -> (-8.3333, 0)
  line L8 (-72, -32.1429) -> (-72, -42.8571)
  line L9 (-72, -42.8571) -> (-75, -42.8571)
  line L10 (-75, -42.8571) -> (-75, -32.1429)
  line L11 (-75, -32.1429) -> (-72, -32.1429)
  line L12 (-3, -10.7143) -> (0, -10.7143)
  line L13 (0, -10.7143) -> (0, -21.4286)
  line L14 (0, -21.4286) -> (-3, -21.4286)
  line L15 (-3, -21.4286) -> (-3, -10.7143)
  line L16 (0, -42.8571) -> (-3, -42.8571)
  line L17 (-3, -42.8571) -> (-3, -32.1429)
  line L18 (-3, -32.1429) -> (0, -32.1429)
  line L19 (0, -32.1429) -> (0, -42.8571)
  line L20 (-66.6667, -72) -> (-58.3333, -72)
  line L21 (-58.3333, -72) -> (-58.3333, -75)
  line L22 (-58.3333, -75) -> (-66.6667, -75)
  line L23 (-66.6667, -75) -> (-66.6667, -72)
  line L24 (-3, -64.2857) -> (-3, -53.5714)
  line L25 (-3, -53.5714) -> (0, -53.5714)
  line L26 (0, -53.5714) -> (0, -64.2857)
  line L27 (0, -64.2857) -> (-3, -64.2857)
  line L28 (-50, -75) -> (-50, -72)
  line L29 (-50, -72) -> (-41.6667, -72)
  line L30 (-41.6667, -72) -> (-41.6667, -75)
  line L31 (-41.6667, -75) -> (-50, -75)
  line L32 (-75, -21.4286) -> (-75, -10.7143)
  line L33 (-75, -10.7143) -> (-72, -10.7143)
  line L34 (-72, -10.7143) -> (-72, -21.4286)
  line L35 (-72, -21.4286) -> (-75, -21.4286)
  line L36 (-33.3333, -72) -> (-25, -72)
  line L37 (-25, -72) -> (-25, -75)
  line L38 (-25, -75) -> (-33.3333, -75)
  line L39 (-33.3333, -75) -> (-33.3333, -72)
  line L40 (-75, -64.2857) -> (-75, -53.5714)
  line L41 (-75, -53.5714) -> (-72, -53.5714)
  line L42 (-72, -53.5714) -> (-72, -64.2857)
  line L43 (-72, -64.2857) -> (-75, -64.2857)
  line L44 (-66.6667, -3) -> (-66.6667, 0)
  line L45 (-66.6667, 0) -> (-58.3333, 0)
  line L46 (-58.3333, 0) -> (-58.3333, -3)
  line L47 (-58.3333, -3) -> (-66.6667, -3)
  line L48 (-41.6667, -3) -> (-50, -3)
  line L49 (-50, -3) -> (-50, 0)
  line L50 (-50, 0) -> (-41.6667, 0)
  line L51 (-41.6667, 0) -> (-41.6667, -3)
  line L52 (-16.6667, -72) -> (-8.3333, -72)
  line L53 (-8.3333, -72) -> (-8.3333, -75)
  line L54 (-8.3333, -75) -> (-16.6667, -75)
  line L55 (-16.6667, -75) -> (-16.6667, -72)
  line L56 (5, -80) -> (5, 5)
  line L57 (5, 5) -> (-80, 5)
  line L58 (-80, 5) -> (-80, -80)
  line L59 (-80, -80) -> (5, -80)
sketch "slide door.dxf" plane through (0, 69, 0) normal (0, -1, 0) x (1, 0, 0) in component "slide door"
  line L0 (38, 24) -> (18, 24)
  arc A0 (18, 34) -> (18, 24) centre (18, 29) ccw
  line L1 (18, 34) -> (38, 34)
  line L2 (38, 34) -> (38, 24)
  line L3 (3, 3) -> (75, 3)
  line L4 (75, 3) -> (75, 78)
  line L5 (75, 78) -> (3, 78)
  line L6 (3, 78) -> (3, 3)
sketch "slider guide.dxf" plane through (0, 66, 0) normal (0, -1, 0) x (1, 0, 0) in component "slider guide"
  line L0 (66.6667, 3) -> (72, 3)
  line L1 (72, 3) -> (72, 8)
  line L2 (72, 8) -> (3, 8)
  line L3 (3, 8) -> (3, 3)
  line L4 (3, 3) -> (8.3333, 3)
  line L5 (8.3333, 3) -> (8.3333, 0)
  line L6 (8.3333, 0) -> (16.6667, 0)
  line L7 (16.6667, 0) -> (16.6667, 3)
  line L8 (16.6667, 3) -> (25, 3)
  line L9 (25, 3) -> (25, 0)
  line L10 (25, 0) -> (33.3333, 0)
  line L11 (33.3333, 0) -> (33.3333, 3)
  line L12 (33.3333, 3) -> (41.6667, 3)
  line L13 (41.6667, 3) -> (41.6667, 0)
  line L14 (41.6667, 0) -> (50, 0)
  line L15 (50, 0) -> (50, 3)
  line L16 (50, 3) -> (58.3333, 3)
  line L17 (58.3333, 3) -> (58.3333, 0)
  line L18 (58.3333, 0) -> (66.6667, 0)
  line L19 (66.6667, 0) -> (66.6667, 3)
sketch "mid panel.dxf" plane through (0, 0, 130) normal (0, 0, 1) x (-1, 0, 0) in component "mid panel"
  line L0 (-31.5, -26.125) -> (-31.5, -53.875)
  line L1 (-31.5, -53.875) -> (-12.5, -53.875)
  line L2 (-12.5, -53.875) -> (-12.5, -63.875)
  line L3 (-12.5, -63.875) -> (-62.5, -63.875)
  line L4 (-62.5, -63.875) -> (-62.5, -53.875)
  line L5 (-62.5, -53.875) -> (-43.5, -53.875)
  line L6 (-43.5, -53.875) -> (-43.5, -26.125)
  line L7 (-43.5, -26.125) -> (-31.5, -26.125)
  line L8 (-75, -52.5) -> (-72, -52.5)
  line L9 (-72, -52.5) -> (-72, -72)
  line L10 (-72, -72) -> (-3, -72)
  line L11 (-3, -72) -> (-3, -52.5)
  line L12 (-3, -52.5) -> (0, -52.5)
  line L13 (0, -52.5) -> (0, -42.8571)
  line L14 (0, -42.8571) -> (-3, -42.8571)
  line L15 (-3, -42.8571) -> (-3, -32.1429)
  line L16 (-3, -32.1429) -> (0, -32.1429)
  line L17 (0, -32.1429) -> (0, -22.5)
  line L18 (0, -22.5) -> (-3, -22.5)
  line L19 (-3, -22.5) -> (-3, -3)
  line L20 (-3, -3) -> (-25, -3)
  line L21 (-25, -3) -> (-25, 0)
  line L22 (-25, 0) -> (-33.3333, 0)
  line L23 (-33.3333, 0) -> (-33.3333, -3)
  line L24 (-33.3333, -3) -> (-41.6667, -3)
  line L25 (-41.6667, -3) -> (-41.6667, 0)
  line L26 (-41.6667, 0) -> (-50, 0)
  line L27 (-50, 0) -> (-50, -3)
  line L28 (-50, -3) -> (-72, -3)
  line L29 (-72, -3) -> (-72, -22.5)
  line L30 (-72, -22.5) -> (-75, -22.5)
  line L31 (-75, -22.5) -> (-75, -32.1429)
  line L32 (-75, -32.1429) -> (-72, -32.1429)
  line L33 (-72, -32.1429) -> (-72, -42.8571)
  line L34 (-72, -42.8571) -> (-75, -42.8571)
  line L35 (-75, -42.8571) -> (-75, -52.5)